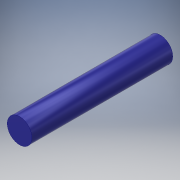
# Autodesk Inventor part: core_b_termination
Saved by Autodesk Inventor 2019 (Build 230136000, 136)
## iProperties
Created: 2021-08-31
Part Number: core_b_termination
Material: Generic
Document SubType Name: Modeling
Designer: zachm
Density: 1 g/cm^3
Appearance: Smooth - Navy
Author: zachm
Autodesk Inventor part; units mm, degrees
ref_plane "YZ Plane" through (0, 0, 0) normal (1, 0, 0) x (0, 1, 0)
ref_plane "XZ Plane" through (0, 0, 0) normal (0, 1, 0) x (-1, 0, 0)
ref_plane "XY Plane" through (0, 0, 0) normal (0, 0, 1) x (1, 0, 0)
sketch "Sketch1" plane through (0, 0, 0) normal (0, 0, 1) x (1, 0, 0)
  circle A0 centre (0, 0) radius 1.75
  dimension "d0" = 3.5
  constraints: 1 centre point, 1 coincident
  measures "d0" diameter of A0
extrude "Extrusion1" add sketch "Sketch1" along normal blind 20
body "Solid1"
